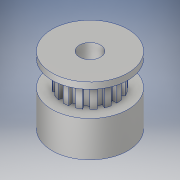
# Autodesk Inventor part: T2.5 16T Pulley
Saved by Autodesk Inventor 2018 (Build 220112000, 112)
## iProperties
Created: 2013-10-02
Part Number: T2.5 16T Pulley
Material: Aluminum 6061
Document SubType Name: Modeling
Designer: Gabriel Smolnycki
Mass: 7.79265 g
Surface Area: 19.9041 cm^2
Volume: 2.88617 cm^3
Density: 2.7 g/cm^3
Appearance: Aluminum - Flat
Sending System: SolidWorks 2017
Last Author: Gabriel Smolnycki
Last Saved: 2017-09-14
Author: Gabriel Smolnycki
Autodesk Inventor part; units mm, degrees
ref_plane "YZ Plane" through (0, 0, 0) normal (1, 0, 0) x (0, 1, 0)
ref_plane "XY Plane" through (0, 0, 0) normal (0, 0, 1) x (1, 0, 0)
ref_plane "Work Plane1" through (0, 16, 0) normal (0, 1, 0) x (-1, 0, 0)
sketch "Sketch1" plane through (0, 16, 0) normal (0, 1, 0) x (-1, 0, 0)
  circle A0 centre (0, 0) radius 9
  constraints: 1 centre point
extrude "Extrusion3" add sketch "Sketch1" against normal blind 16
ref_plane "Work Plane2" through (0, 14.5, 0) normal (0, 1, 0) x (-1, 0, 0)
sketch "Sketch2" plane through (0, 14.5, 0) normal (0, 1, 0) x (-1, 0, 0)
  arc A0 (4.4703, 2.987) -> (3.8017, 3.8017) centre (0, 0) ccw
  line L0 (2.987, -4.4703) -> (3.5426, -5.3018)
  arc A1 (-5.8911, -2.4402) -> (-5.3018, -3.5426) centre (0, 0) ccw
  line L1 (-2.4402, 5.8911) -> (-2.0575, 4.9672)
  line L2 (2.987, 4.4703) -> (3.5426, 5.3018)
  arc A2 (4.5088, -4.5088) -> (5.3018, -3.5426) centre (0, 0) ccw
  line L3 (-4.5088, -4.5088) -> (-3.8017, -3.8017)
  arc A3 (-2.987, 4.4703) -> (-3.8017, 3.8017) centre (0, 0) ccw
  arc A4 (2.4402, 5.8911) -> (1.244, 6.2539) centre (0, 0) ccw
  line L4 (5.8911, -2.4402) -> (4.9672, -2.0575)
  arc A5 (-2.987, -4.4703) -> (-2.0575, -4.9672) centre (0, 0) ccw
  line L5 (-4.4703, 2.987) -> (-5.3018, 3.5426)
  line L6 (0, 6.3764) -> (0, 5.3764)
  arc A6 (5.2731, -1.0489) -> (5.3764, 0) centre (0, 0) ccw
  line L7 (-1.0489, -5.2731) -> (-1.244, -6.2539)
  arc A7 (-5.8911, 2.4402) -> (-6.2539, 1.244) centre (0, 0) ccw
  line L8 (5.2731, 1.0489) -> (6.2539, 1.244)
  arc A8 (0, -6.3764) -> (1.244, -6.2539) centre (0, 0) ccw
  line L9 (-6.3764, 0) -> (-5.3764, 0)
  arc A9 (5.8911, 2.4402) -> (5.3018, 3.5426) centre (0, 0) ccw
  line L10 (2.4402, -5.8911) -> (2.0575, -4.9672)
  arc A10 (-5.2731, -1.0489) -> (-4.9672, -2.0575) centre (0, 0) ccw
  line L11 (-1.0489, 5.2731) -> (-1.244, 6.2539)
  line L12 (4.5088, 4.5088) -> (3.8017, 3.8017)
  arc A11 (2.987, -4.4703) -> (3.8017, -3.8017) centre (0, 0) ccw
  line L13 (-4.4703, -2.987) -> (-5.3018, -3.5426)
  arc A12 (-2.4402, 5.8911) -> (-3.5426, 5.3018) centre (0, 0) ccw
  arc A13 (2.987, 4.4703) -> (2.0575, 4.9672) centre (0, 0) ccw
  line L14 (4.4703, -2.987) -> (5.3018, -3.5426)
  arc A14 (-4.5088, -4.5088) -> (-3.5426, -5.3018) centre (0, 0) ccw
  line L15 (-4.5088, 4.5088) -> (-3.8017, 3.8017)
  line L16 (1.0489, 5.2731) -> (1.244, 6.2539)
  arc A15 (5.8911, -2.4402) -> (6.2539, -1.244) centre (0, 0) ccw
  line L17 (-2.4402, -5.8911) -> (-2.0575, -4.9672)
  arc A16 (-4.4703, 2.987) -> (-4.9672, 2.0575) centre (0, 0) ccw
  arc A17 (0, 6.3764) -> (-1.244, 6.2539) centre (0, 0) ccw
  line L18 (6.3764, 0) -> (5.3764, 0)
  arc A18 (-1.0489, -5.2731) -> (0, -5.3764) centre (0, 0) ccw
  line L19 (-5.2731, 1.0489) -> (-6.2539, 1.244)
  arc A19 (5.2731, 1.0489) -> (4.9672, 2.0575) centre (0, 0) ccw
  line L20 (1.0489, -5.2731) -> (1.244, -6.2539)
  arc A20 (-6.3764, 0) -> (-6.2539, -1.244) centre (0, 0) ccw
  line L21 (4.4703, 2.987) -> (5.3018, 3.5426)
  arc A21 (2.4402, -5.8911) -> (3.5426, -5.3018) centre (0, 0) ccw
  line L22 (-5.8911, -2.4402) -> (-4.9672, -2.0575)
  arc A22 (-1.0489, 5.2731) -> (-2.0575, 4.9672) centre (0, 0) ccw
  arc A23 (4.5088, 4.5088) -> (3.5426, 5.3018) centre (0, 0) ccw
  line L23 (4.5088, -4.5088) -> (3.8017, -3.8017)
  arc A24 (-4.4703, -2.987) -> (-3.8017, -3.8017) centre (0, 0) ccw
  line L24 (-2.987, 4.4703) -> (-3.5426, 5.3018)
  line L25 (2.4402, 5.8911) -> (2.0575, 4.9672)
  arc A25 (4.4703, -2.987) -> (4.9672, -2.0575) centre (0, 0) ccw
  line L26 (-2.987, -4.4703) -> (-3.5426, -5.3018)
  arc A26 (-4.5088, 4.5088) -> (-5.3018, 3.5426) centre (0, 0) ccw
  arc A27 (1.0489, 5.2731) -> (0, 5.3764) centre (0, 0) ccw
  line L27 (5.2731, -1.0489) -> (6.2539, -1.244)
  arc A28 (-2.4402, -5.8911) -> (-1.244, -6.2539) centre (0, 0) ccw
  line L28 (-5.8911, 2.4402) -> (-4.9672, 2.0575)
  circle A29 centre (0, 0) radius 9
  arc A30 (6.3764, 0) -> (6.2539, 1.244) centre (0, 0) ccw
  line L29 (0, -6.3764) -> (0, -5.3764)
  arc A31 (-5.2731, 1.0489) -> (-5.3764, 0) centre (0, 0) ccw
  line L30 (5.8911, 2.4402) -> (4.9672, 2.0575)
  arc A32 (1.0489, -5.2731) -> (2.0575, -4.9672) centre (0, 0) ccw
  line L31 (-5.2731, -1.0489) -> (-6.2539, -1.244)
  constraints: 64 end point, 64 point on circle, 33 centre point, 31 equal length, 16 collinear, 7 perpendicular, 2 horizontal, 2 vertical
extrude "Extrusion2" cut sketch "Sketch2" against normal blind 6
sketch "Sketch3" plane through (0, 0, 0) normal (0, 1, 0) x (-1, 0, 0)
  circle A0 centre (0, 0) radius 2.5
  constraints: 1 centre point
extrude "Extrusion1" cut sketch "Sketch3" along normal blind 16
body "Solid3"
